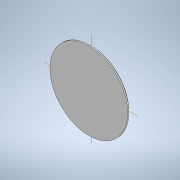
# Autodesk Inventor part: half_wheel_string
Saved by Autodesk Inventor 2022 (Build 260153000, 153)
## iProperties
Created: 2021-11-30
Part Number: half_wheel_string
Material: Generic
Document SubType Name: Modeling
Designer: verve
Density: 1 g/cm^3
Appearance: Default
Author: verve
Autodesk Inventor part; units mm, degrees
ref_plane "YZ Plane" through (0, 0, 0) normal (1, 0, 0) x (0, 1, 0)
ref_plane "XZ Plane" through (0, 0, 0) normal (0, 1, 0) x (-1, 0, 0)
sketch "Sketch3" plane through (0, 0, 0) normal (1, 0, 0) x (0, 1, 0)
  line L0 (0, 0) -> (50.85, 0)
  line L1 (50.85, 0) -> (50.85, 3)
  line L2 (50.85, 3) -> (0, 3)
  line L3 (0, 3) -> (0, 0)
  dimension "d3" = 50.85
  dimension "d4" = 3
  constraints: 8 end point, 2 parallel, 1 horizontal, 1 perpendicular
  measures "d3" distance of L2.end L1.end
  measures "d4" distance of L0.end L1.end
revolve "Revolution2" add sketch "Sketch3" angle 360 about axis through (0, 0, 3) along (0, 0, -1)
ref_plane "Work Plane2" through (0, 0, 1.5) normal (0, 0, -1) x (-1, 0, 0)
sketch "Sketch4" plane through (0, 0, 1.5) normal (0, 0, -1) x (-1, 0, 0)
  circle A0 centre (0, 0) radius 50.85 projected
  circle A1 centre (0, 50.85) radius 5.1464
  circle A2 centre (0, 50.85) radius 7.5
  point P0 (-7.4796, 50.2969)
  point P1 (7.4796, 50.2969)
  point P2 (5.1398, 50.5896)
  point P3 (-5.1398, 50.5896)
  dimension "d6" = 15
  constraints: 2 centre point, 1 coincident, 2 other
  measures "d6" diameter of A2
extrude "Extrusion1" cut sketch "Sketch4" along normal blind 10 contours A2 A0 A1 picked at (5.9615, 47.8508)
fillet "Fillet1" radius 1.5 3 edges at (0, -50.85, 0) (2.5732, 50.7849, 0) (-2.5732, 50.7849, 0) inverted yes
body "Solid2"
